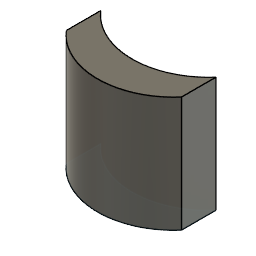
Motor Mount Slide (Autodesk Fusion 360 design; units mm, degrees)
part number: 2026-05-27-13-45-06-740
Autodesk Fusion 360 part; units mm, degrees
sketch "Sketch1" plane through (0, 0, 0) normal (0, 1, 0) x (1, 0, 0)
  line L0 (0, -3) -> (0, 0)
  line L1 (10, -3) -> (10, 0)
  arc A0 (0, 0) -> (10, 0) centre (5, 4.3372) ccw
  arc A1 (0, -3) -> (10, -3) centre (5, 1.3372) ccw
  dimension "d2" = 10
  dimension "d3" = 3
  dimension "d4" = 6.619
  constraint vertical L0
  constraint vertical L1
  constraint equal L0 L1
  constraint equal A0 A1
  constraint horizontal L0.end L1.end
  constraint coincident L0.end A0.start
  measures "d2" distance of L0 L1
  measures "d3" distance of L1.start L1.end
  measures "d4" radius of A0
extrude "Extrude1" add sketch "Sketch1" along normal blind 10
sketch "Sketch2" plane through (0, 0, 0) normal (0, -1, 0) x (1, 0, 0)
  line L0 (0, 3) -> (0, 0)
  arc A0 (10, 0) -> (0, 0) centre (5, -4.3372) ccw
  line L1 (10, 0) -> (10, 3)
  arc A1 (10, 3) -> (0, 3) centre (5, -1.3372) ccw
